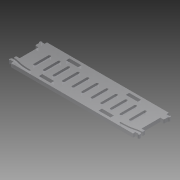
# Autodesk Inventor part: LeftPanel
Saved by Autodesk Inventor 2015 SP1 (Build 190203100, 203)
## iProperties
Created: 2015-01-22
Part Number: LeftPanel
Material: Acrylic, Clear
Document SubType Name: Modeling
Designer: Patrick
Density: 1.19 g/cm^3
Appearance: Transparent - Clear
Author: Patrick
Autodesk Inventor part; units mm, degrees
ref_plane "YZ Plane" through (0, 0, 0) normal (1, 0, 0) x (0, 1, 0)
ref_plane "XZ Plane" through (0, 0, 0) normal (0, 1, 0) x (-1, 0, 0)
ref_plane "XY Plane" through (0, 0, 0) normal (0, 0, 1) x (1, 0, 0)
sketch "Sketch1" plane through (0, 0, 0) normal (0, 0, 1) x (1, 0, 0)
  line L0 (-51, 15) -> (51, 15)
  line L1 (51, 15) -> (51, -15)
  line L2 (51, -15) -> (-51, -15)
  line L3 (-51, -15) -> (-51, 15)
  line L4 (-51, 15) -> (51, -15) construction
  line L5 (51, 15) -> (-51, -15) construction
  point P0 (0, 0)
  dimension "d0" = 102
  dimension "d1" = 30
  constraints: 12 end point, 2 midpoint, 2 parallel, 1 horizontal, 1 perpendicular
  measures "d0" distance of L1.end L2.end
  measures "d1" distance of L0.end L1.end
extrude "Extrusion1" add sketch "Sketch1" along normal blind 3
sketch "Sketch2" plane through (0, 0, 0) normal (0, 0, -1) x (-1, 0, 0)
  line L0 (-51, 13) -> (-53.87, 13)
  line L1 (-53.87, 13) -> (-53.87, 7.87)
  line L2 (-53.87, 7.87) -> (-51, 7.87)
  line L3 (-51, 7.87) -> (-51, 13)
  line L4 (-50, -13) -> (-53.87, -13)
  line L5 (-53.87, -13) -> (-53.87, -7.87)
  line L6 (-53.87, -7.87) -> (-50, -7.87)
  line L7 (-50, -7.87) -> (-50, -13)
  arc A0 (-53.87, 13.8784) -> (-53.87, 11.1216) centre (-53, 12.5) ccw
  arc A1 (-53.87, -11.1216) -> (-53.87, -13.8784) centre (-53, -12.5) ccw
  line L8 (-53.87, 13.8784) -> (-53.87, 11.1216)
  line L9 (-53.87, -11.1216) -> (-53.87, -13.8784)
  line L10 (-51, 15) -> (-51, -15) projected
  line L11 (51, 15) -> (-51, 15) projected
  line L12 (-51, -15) -> (51, -15) projected
  point P0 (0, 0)
  dimension "d15" = 2.87
  dimension "d16" = 5.13
  dimension "d17" = 5.13
  dimension "d18" = 1.63
  dimension "d19" = 1.63
  dimension "d20" = 0.5
  dimension "d21" = 0.5
  dimension "d22" = 2
  dimension "d23" = 2
  constraints: 20 end point, 4 parallel, 4 point on circle, 2 centre point, 2 collinear, 2 horizontal, 2 perpendicular, 2 point on line, 2 vertical
  measures "d15" distance of L3.start L1.end
  measures "d16" distance of L1.end L0.end
  measures "d17" distance of L4.end L5.end
  measures "d18" radius of A0
  measures "d19" radius of A1
  measures "d20" distance from line of L0 A0.centre
  measures "d21" distance from line of L4 A1.centre
  measures "d22" distance between parallel lines of L0 L11
  measures "d23" distance between parallel lines of L4 L12
extrude "Extrusion2" add sketch "Sketch2" against normal blind 3
mirror "Mirror1" about plane through (0, 0, 0) normal (1, 0, 0) of "Extrusion2"
sketch "Sketch3" plane through (0, 0, 0) normal (0, 0, -1) x (-1, 0, 0)
  line L0 (29.985, -12.82) -> (20.015, -12.82)
  line L1 (20.015, -12.82) -> (20.015, -10)
  line L2 (20.015, -10) -> (29.985, -10)
  line L3 (29.985, -10) -> (29.985, -12.82)
  line L4 (29.985, -12.82) -> (20.015, -10) construction
  line L5 (20.015, -12.82) -> (29.985, -10) construction
  line L6 (29.985, 10) -> (20.015, 10)
  line L7 (20.015, 10) -> (20.015, 12.82)
  line L8 (20.015, 12.82) -> (29.985, 12.82)
  line L9 (29.985, 12.82) -> (29.985, 10)
  line L10 (29.985, 10) -> (20.015, 12.82) construction
  line L11 (20.015, 10) -> (29.985, 12.82) construction
  point P0 (0, 0)
  point P1 (25, -11.41)
  point P2 (25, 11.41)
  dimension "d26" = 9.97
  dimension "d27" = 2.82
  dimension "d29" = 25
  dimension "d31" = 10
  dimension "d32" = 10
  constraints: 24 end point, 4 midpoint, 4 parallel, 2 equal length, 2 horizontal, 2 perpendicular, 1 point on line
  measures "d26" distance of L1.end L2.end
  measures "d27" distance of L0.end L1.end
  measures "d29" horizontal distance of point (25, -11.41) point (0, 0)
  measures "d31" distance from line of L2 point (0, 0)
  measures "d32" distance from line of L6 point (0, 0)
extrude "Extrusion3" cut sketch "Sketch3" against normal through all
mirror "Mirror2" about plane through (0, 0, 0) normal (1, 0, 0) of "Extrusion3"
sketch "Sketch4" plane through (0, 0, 3) normal (0, 0, 1) x (1, 0, 0)
  line L0 (-51, -15) -> (51, -15) projected
  line L1 (-53.87, -11.1216) -> (-48.4188, -11.1216) construction
  line L2 (-48.4188, -11.1216) -> (-48.4188, -13) construction
  line L3 (-48.4188, -13) -> (-38, -13) construction
  spline S0 degree 3 poles (-53.87, -11.1216) (-48.4188, -11.1216) (-48.4188, -13) (-38, -13) knots 1 1 1 1 2 2 2 2
  line L4 (-53.87, -9.9216) -> (-48.4188, -9.9216) construction
  line L5 (-48.4188, -9.9216) -> (-48.4188, -11.8) construction
  line L6 (-48.4188, -11.8) -> (-38, -11.8) construction
  spline S1 degree 3 poles (-53.87, -9.9216) (-48.4188, -9.9216) (-48.4188, -11.8) (-38, -11.8) knots 1 1 1 1 2 2 2 2
  arc A0 (-38, -13) -> (-38, -11.8) centre (-38, -12.4) ccw
  line L7 (-53.87, -11.1216) -> (-53.87, -9.9216)
  line L8 (-53.87, -7.87) -> (-53.87, -11.1216) projected
  point P0 (0, 0)
  dimension "d40" = 2
  dimension "d41" = 1.2
  dimension "d44" = 0.6
  constraints: 4 horizontal, 2 end point, 2 point on circle, 2 tangent, 2 vertical, 1 centre point, 1 collinear, 6 other
  measures "d40" distance from line of L0 L3.end
  measures "d41" distance of L1.start L4.start
  measures "d44" radius of A0
extrude "Extrusion5" cut sketch "Sketch4" against normal through all
mirror "Mirror4" about plane through (0, 0, 0) normal (1, 0, 0) of "Extrusion5"
fillet "Fillet1" radius 1 1 edges at (53.87, 7.87, 1.5)
fillet "Fillet2" radius 1 1 edges at (-53.87, 7.87, 1.5)
sketch "Sketch5" plane through (0, 0, 3) normal (0, 0, 1) x (1, 0, 0)
  line L0 (0, -6) -> (0, 6) construction
  line L1 (1, -6) -> (1, 6)
  line L2 (-1, 6) -> (-1, -6)
  arc A0 (-1, -6) -> (1, -6) centre (0, -6) ccw
  arc A1 (1, 6) -> (-1, 6) centre (0, 6) ccw
  point P0 (0, 0)
  dimension "d47" = 6
  dimension "d48" = 2
  constraints: 8 end point, 4 point on circle, 4 tangent, 2 centre point, 1 midpoint, 1 parallel, 1 vertical
  measures "d47" distance of point (0, 0) L0.end
  measures "d48" diameter of A1
extrude "Extrusion6" cut sketch "Sketch5" against normal blind 10
pattern_linear "Rectangular Pattern1" count 11 spacing 8 along (-1, 0, 0) of "Extrusion6" first direction both ways yes
equation "\"d17\" = d16"
equation "\"d19\" = d18"
equation "\"d21\" = d20"
equation "\"d23\" = d22"
equation "\"d32\" = d31"
equation "\"d44\" = 0.5 * d41"
equation "\"kerf\" = 0.13"
body "Solid1"
